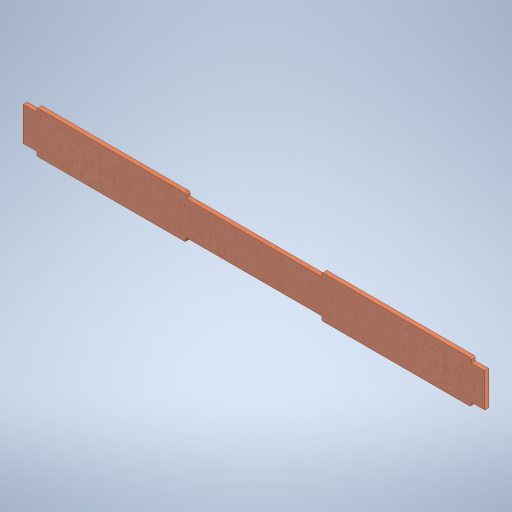
# Autodesk Inventor part: ConectorPared
Saved by Autodesk Inventor 2024 (Build 280153000, 153)
## iProperties
Created: 2023-11-02
Part Number: ConectorPared
Material: Generic
Document SubType Name: Modeling
Designer: fredy
Density: 1 g/cm^3
Appearance: Walnut - Natural Polished
Author: fredy
Autodesk Inventor part; units mm, degrees
ref_plane "YZ Plane" through (0, 0, 0) normal (1, 0, 0) x (0, 1, 0)
ref_plane "XZ Plane" through (0, 0, 0) normal (0, 1, 0) x (-1, 0, 0)
ref_plane "XY Plane" through (0, 0, 0) normal (0, 0, 1) x (1, 0, 0)
sketch "Sketch1" plane through (0, 0, 0) normal (0, 0, 1) x (1, 0, 0)
  line L0 (-170, 0) -> (-170, 12.5)
  line L1 (-170, 12.5) -> (-160, 12.5)
  line L2 (-160, 12.5) -> (-160, 15.5)
  line L3 (-160, 15.5) -> (-50, 15.5)
  line L4 (-50, 15.5) -> (-50, 12.5)
  line L5 (-50, 12.5) -> (0, 12.5)
  line L6 (-238, 0) -> (238, 0) projected
  line L7 (-170, 0) -> (-170, -12.5)
  line L8 (-170, -12.5) -> (-160, -12.5)
  line L9 (-160, -12.5) -> (-160, -15.5)
  line L10 (-160, -15.5) -> (-50, -15.5)
  line L11 (-50, -15.5) -> (-50, -12.5)
  line L12 (-50, -12.5) -> (0, -12.5)
  line L13 (0, -21.7) -> (0, 21.7) projected
  line L14 (170, 0) -> (170, 12.5)
  line L15 (170, 12.5) -> (160, 12.5)
  line L16 (160, 12.5) -> (160, 15.5)
  line L17 (160, 15.5) -> (50, 15.5)
  line L18 (50, 15.5) -> (50, 12.5)
  line L19 (50, 12.5) -> (0, 12.5)
  line L20 (170, 0) -> (170, -12.5)
  line L21 (170, -12.5) -> (160, -12.5)
  line L22 (160, -12.5) -> (160, -15.5)
  line L23 (160, -15.5) -> (50, -15.5)
  line L24 (50, -15.5) -> (50, -12.5)
  line L25 (50, -12.5) -> (0, -12.5)
  point P0 (0, 0)
  point P1 (50, 14)
  point P2 (-50, 14)
  point P3 (-165, -12.5)
  point P4 (-165, 12.5)
  dimension "d0" = 3
  dimension "d2" = 100
  dimension "d3" = 10
  dimension "d4" = 110
  dimension "d5" = 25
  constraints: 48 end point, 17 symmetric about line, 9 point on line, 4 midpoint, 4 perpendicular, 1 vertical
  measures "d0" distance of L2.end L1.end
  measures "d2" distance of point (50, 14) point (-50, 14)
  measures "d3" distance of L0.end L1.end
  measures "d4" distance of L2.end L3.end
  measures "d5" distance of point (-165, -12.5) point (-165, 12.5)
extrude "Extrusion1" add sketch "Sketch1" along normal blind 3
fillet "Fillet1" radius 1 8 edges at (-160, 15.5, 1.5) (-50, 15.5, 1.5) (50, 15.5, 1.5) (160, 15.5, 1.5) (160, -15.5, 1.5) (50, -15.5, 1.5) (-50, -15.5, 1.5) (-160, -15.5, 1.5)
body "Solid1"
